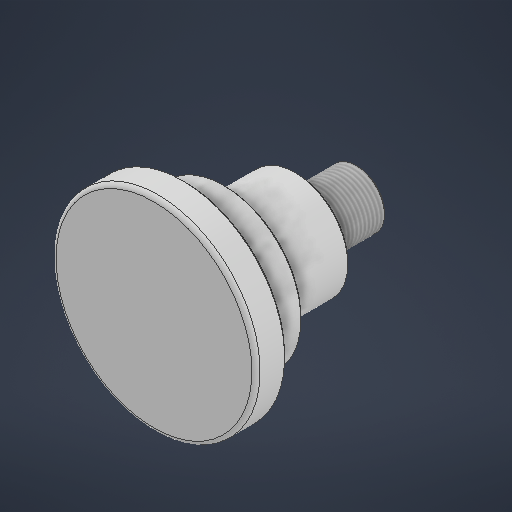
# Autodesk Inventor part: Part4
Saved by Autodesk Inventor 2026 (Build 300175050, 175E)
## iProperties
Created: 2026-03-26
Part Number: Part4
Material: Generic
Document SubType Name: Modeling
Designer: Administrator
Density: 1 g/cm^3
Appearance: Default
Author: Administrator
Autodesk Inventor part; units mm, degrees
ref_plane "YZ Plane" through (0, 0, 0) normal (1, 0, 0) x (0, 1, 0)
ref_plane "XZ Plane" through (0, 0, 0) normal (0, 1, 0) x (-1, 0, 0)
ref_plane "XY Plane" through (0, 0, 0) normal (0, 0, 1) x (1, 0, 0)
sketch "Sketch1" plane through (0, 0, 0) normal (1, 0, 0) x (0, 1, 0)
  line L0 (0, 0) -> (0, -100)
  line L1 (0, -100) -> (14, -100)
  line L2 (14, -100) -> (14, -70)
  line L3 (14, -70) -> (26, -70)
  line L4 (26, -70) -> (26, -35)
  line L5 (26, -35) -> (38, -35)
  line L6 (38, -35) -> (38, -15)
  line L7 (38, -15) -> (50, -15)
  line L8 (50, -15) -> (50, 0)
  line L9 (50, 0) -> (0, 0)
  dimension "d0" = 100
  dimension "d1" = 15
  dimension "d2" = 20
  dimension "d3" = 35
  dimension "d4" = 50
  dimension "d5" = 12
  dimension "d6" = 12
  dimension "d7" = 12
  dimension "d8" = 28
  dimension "d9" = 52
  dimension "d10" = 76
  dimension "d11" = 100
  constraints: 20 end point, 9 perpendicular, 1 vertical
  measures "d0" distance of L0.start L0.end
  measures "d1" distance of L7.end L8.end
  measures "d2" distance of L5.end L6.end
  measures "d3" distance of L3.end L4.end
  measures "d4" distance of L8.end L0.start
  measures "d5" distance of L4.end L5.end
  measures "d6" distance of L6.end L7.end
  measures "d7" distance of L2.end L3.end
  measures "d8" diameter of L2 L0
  measures "d9" diameter of L4 L0
  measures "d10" diameter of L6 L0
  measures "d11" diameter of L8 L0
revolve "Revolution1" add sketch "Sketch1" angle 360 about axis through (0, 0, 0) along (0, 0, -1)
chamfer "Chamfer1" distance 1 angle 45 1 edges at (0, -14, -100)
chamfer "Chamfer2" distance 1 angle 45 1 edges at (0, -26, -70)
chamfer "Chamfer3" distance 1 angle 45 1 edges at (0, -38, -35)
chamfer "Chamfer4" distance 1 angle 45 1 edges at (0, -50, -15)
fillet "Fillet1" radius 2 1 edges at (0, -14, -70)
fillet "Fillet2" radius 2 1 edges at (0, -26, -35)
fillet "Fillet3" radius 2 1 edges at (0, -38, -15)
fillet "Fillet4" radius 2 1 edges at (0, -50, 0)
thread "Thread1" size "M28x2" class "6g" standard "ANSI Metric M Profile" full length
body "Solid1"
